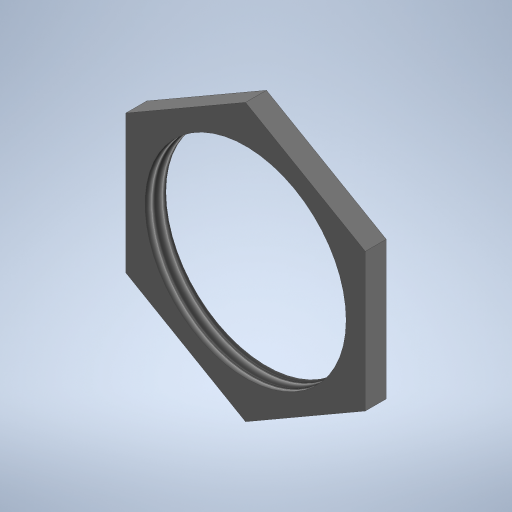
# Autodesk Inventor part: USB NUT
Saved by Autodesk Inventor 2023 (Build 270158000, 158)
## iProperties
Created: 2023-04-24
Part Number: USB NUT
Material: Generic
Document SubType Name: Modeling
Designer: Louis
Density: 1 g/cm^3
Appearance: Default
Author: Louis
Autodesk Inventor part; units mm, degrees
ref_plane "YZ Plane" through (0, 0, 0) normal (1, 0, 0) x (0, 1, 0)
ref_plane "XZ Plane" through (0, 0, 0) normal (0, 1, 0) x (-1, 0, 0)
ref_plane "XY Plane" through (0, 0, 0) normal (0, 0, 1) x (1, 0, 0)
sketch "Sketch1" plane through (0, 0, 0) normal (0, 0, 1) x (1, 0, 0)
  line L0 (0, 16.5122) -> (14.3, 8.2561)
  line L1 (14.3, 8.2561) -> (14.3, -8.2561)
  line L2 (14.3, -8.2561) -> (0, -16.5122)
  line L3 (0, -16.5122) -> (-14.3, -8.2561)
  line L4 (-14.3, -8.2561) -> (-14.3, 8.2561)
  line L5 (-14.3, 8.2561) -> (0, 16.5122)
  point P0 (0, 0)
  point P1 (0, 0)
  dimension "d0" = 28.6
  constraints: 12 end point, 1 coincident, 13 other
  measures "d0" distance between parallel lines of L2 L5
extrude "Extrusion1" add sketch "Sketch1" along normal blind 2.5
sketch "Sketch2" plane through (0, 0, 2.5) normal (0, 0, 1) x (1, 0, 0)
  point P0 (0, 0)
hole "Hole1" at (0, 0, 2.5) direction (0, 0, -1) diameter 24.0284 end through all thread size "1-20 UNEF" class "2B" standard "ANSI Unified Screw Threads"
body "Solid1"
